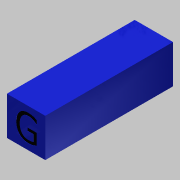
# Autodesk Inventor part: Container 2 2 5 generic
Saved by Autodesk Inventor 2015 (Build 190159000, 159)
## iProperties
Created: 2015-03-07
Part Number: Container 2 2 5 generic
Material: Generic
Document SubType Name: Modeling
Designer: Vukica
Density: 1 g/cm^3
Appearance: Blue - Wall Paint - Glossy
Author: Vukica
Autodesk Inventor part; units mm, degrees
ref_plane "YZ Plane" through (0, 0, 0) normal (1, 0, 0) x (0, 1, 0)
ref_plane "XZ Plane" through (0, 0, 0) normal (0, 1, 0) x (-1, 0, 0)
ref_plane "XY Plane" through (0, 0, 0) normal (0, 0, 1) x (1, 0, 0)
sketch "Sketch1" plane through (0, 0, 0) normal (0, 0, 1) x (1, 0, 0)
  line L0 (0, 0) -> (38.1, 0)
  line L1 (38.1, 0) -> (38.1, 38.1)
  line L2 (38.1, 38.1) -> (0, 38.1)
  line L3 (0, 38.1) -> (0, 0)
  dimension "d0" = 38.1
  dimension "d1" = 38.1
  constraints: 8 end point, 2 parallel, 1 horizontal, 1 perpendicular
  measures "d0" distance of L1.end L2.end
  measures "d1" distance of L2.end L0.start
extrude "Extrusion1" add sketch "Sketch1" along normal blind 127
sketch "Sketch2" plane through (0, 0, 127) normal (0, 0, 1) x (1, 0, 0)
  line L0 (8.0198, 32.2387) -> (54.4149, 32.2387) construction
  line L1 (54.4149, 32.2387) -> (54.4149, -0.3861) construction
  line L2 (54.4149, -0.3861) -> (8.0198, -0.3861) construction
  line L3 (8.0198, -0.3861) -> (8.0198, 32.2387) construction
  spline S0 degree 2 poles (21.2344, 5.8919) (18.5379, 5.8919) (14.0713, 7.5385) (12.4658, 9.2058) knots 0 0 0 1 2 2 2
  spline S1 degree 2 poles (12.4658, 9.2058) (10.8603, 10.8936) (9.1519, 15.8748) (9.1519, 19.1064) knots 0 0 0 1 2 2 2
  spline S2 degree 2 poles (9.1519, 19.1064) (9.1519, 22.1734) (10.8809, 27.0311) (12.4864, 28.7601) knots 0 0 0 1 2 2 2
  spline S3 degree 2 poles (12.4864, 28.7601) (14.0301, 30.4273) (18.5585, 32.2387) (21.2549, 32.2387) knots 0 0 0 1 2 2 2
  spline S4 degree 2 poles (21.2549, 32.2387) (22.5517, 32.2387) (24.8982, 31.8682) (25.9686, 31.5389) knots 0 0 0 1 2 2 2
  spline S5 degree 2 poles (25.9686, 31.5389) (26.8331, 31.2919) (28.9326, 30.3862) (29.5707, 30.0568) knots 0 0 0 1 2 2 2
  line L4 (29.5707, 30.0568) -> (29.5707, 25.9813)
  line L5 (29.5707, 25.9813) -> (29.2825, 25.9813)
  spline S6 degree 2 poles (29.2825, 25.9813) (28.6444, 26.5371) (27.3065, 27.5457) (26.0715, 28.122) knots 0 0 0 1 2 2 2
  spline S7 degree 2 poles (26.0715, 28.122) (25.0423, 28.6366) (22.387, 29.3158) (20.8639, 29.3158) knots 0 0 0 1 2 2 2
  spline S8 degree 2 poles (20.8639, 29.3158) (17.2, 29.3158) (12.6716, 23.7995) (12.6716, 19.2094) knots 0 0 0 1 2 2 2
  spline S9 degree 2 poles (12.6716, 19.2094) (12.6716, 16.657) (13.8655, 12.8285) (14.9976, 11.5111) knots 0 0 0 1 2 2 2
  spline S10 degree 2 poles (14.9976, 11.5111) (16.0885, 10.1938) (19.176, 8.8147) (21.1109, 8.8147) knots 0 0 0 1 2 2 2
  spline S11 degree 2 poles (21.1109, 8.8147) (22.5311, 8.8147) (25.3716, 9.2264) (26.3391, 9.638) knots 0 0 0 1 2 2 2
  line L6 (26.3391, 9.638) -> (26.3391, 16.2042)
  line L7 (26.3391, 16.2042) -> (20.4522, 16.2042)
  line L8 (20.4522, 16.2042) -> (20.4522, 19.1682)
  line L9 (20.4522, 19.1682) -> (29.6736, 19.1682)
  line L10 (29.6736, 19.1682) -> (29.6736, 8.0737)
  spline S12 degree 2 poles (29.6736, 8.0737) (29.0355, 7.7855) (26.8536, 6.9004) (25.9274, 6.6329) knots 0 0 0 1 2 2 2
  spline S13 degree 2 poles (25.9274, 6.6329) (24.6718, 6.2624) (22.6546, 5.8919) (21.2344, 5.8919) knots 0 0 0 1 2 2 2
  point P0 (0, 0)
  constraints: 2 other
extrude "Extrusion3" cut sketch "Sketch2" against normal blind 0.254
equation "\"d1\" = d0"
body "Solid1"
